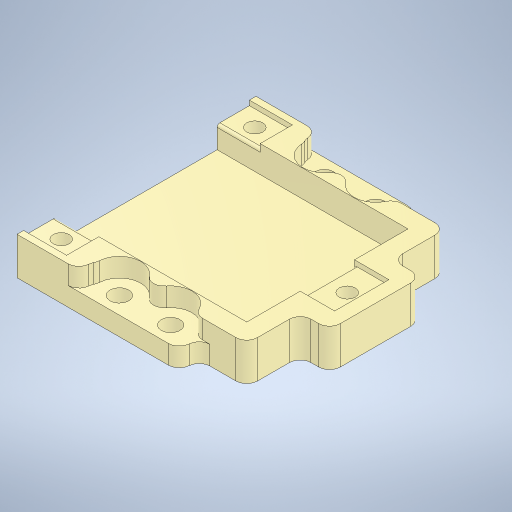
# Autodesk Inventor part: Servo Support
Saved by Autodesk Inventor 2023.2 (Build 272271000, 271)
## iProperties
Created: 2024-01-22
Part Number: Servo Support
Material: Nylon 6/6
Document SubType Name: Modeling
Designer: Nathan Cai
Density: 1.13 g/cm^3
Appearance: Nylon 6
Author: Nathan Cai
Autodesk Inventor part; units mm, degrees
ref_plane "YZ Plane" through (0, 0, 0) normal (1, 0, 0) x (0, 1, 0)
ref_plane "XZ Plane" through (0, 0, 0) normal (0, 1, 0) x (-1, 0, 0)
ref_plane "XY Plane" through (0, 0, 0) normal (0, 0, 1) x (1, 0, 0)
sketch "Sketch8" plane through (0, 0, 0) normal (0, 1, 0) x (-1, 0, 0)
  line L0 (-17.75, 15) -> (17.75, 15)
  line L1 (17.75, 15) -> (17.75, -15)
  line L2 (17.75, -15) -> (-17.75, -15)
  line L3 (-17.75, -15) -> (-17.75, 15)
  line L4 (-17.75, 15) -> (17.75, -15) construction
  line L5 (17.75, 15) -> (-17.75, -15) construction
  line L6 (17.75, 0) -> (-17.75, 0) construction
  line L7 (17.75, 21) -> (9.75, 21)
  line L8 (9.75, 21) -> (9.75, -21)
  line L9 (9.75, -21) -> (17.75, -21)
  line L10 (17.75, -21) -> (17.75, 21)
  line L11 (17.75, 21) -> (9.75, -21) construction
  line L12 (9.75, 21) -> (17.75, -21) construction
  line L13 (13.75, 21) -> (13.75, -21) construction
  circle A0 centre (13.75, 18) radius 1.5
  circle A1 centre (13.75, -18) radius 1.5
  line L14 (-24.15, 5.05) -> (-17.75, 5.05)
  line L15 (-17.75, 5.05) -> (-17.75, -5.05)
  line L16 (-17.75, -5.05) -> (-24.15, -5.05)
  line L17 (-24.15, -5.05) -> (-24.15, 5.05)
  line L18 (-24.15, 5.05) -> (-17.75, -5.05) construction
  line L19 (-17.75, 5.05) -> (-24.15, -5.05) construction
  circle A2 centre (-21.45, 0) radius 1.5
  line L20 (27.275, 14.4) -> (17.75, 14.4)
  line L21 (17.75, 14.4) -> (17.75, 2.4)
  line L22 (17.75, 2.4) -> (27.275, 2.4)
  line L23 (27.275, 2.4) -> (27.275, 14.4)
  line L24 (27.275, 14.4) -> (17.75, 2.4) construction
  line L25 (17.75, 14.4) -> (27.275, 2.4) construction
  line L26 (-26.7, 22.225) -> (17.75, 22.225)
  line L27 (17.75, 22.225) -> (17.75, -22.225)
  line L28 (17.75, -22.225) -> (-26.7, -22.225)
  line L29 (-26.7, -22.225) -> (-26.7, 22.225)
  line L30 (-26.7, 22.225) -> (17.75, -22.225) construction
  line L31 (17.75, 22.225) -> (-26.7, -22.225) construction
  point P0 (0, 0)
  point P1 (13.75, 0)
  point P2 (-20.95, 0)
  point P3 (22.5125, 8.4)
  point P4 (-4.475, 0)
  point P5 (9.75, -15)
  point P6 (9.75, 15)
  dimension "d120" = 35.5
  dimension "d121" = 30
  dimension "d122" = 8
  dimension "d123" = 42
  dimension "d124" = 3
  dimension "d126" = 41.9
  dimension "d127" = 10.1
  dimension "d128" = 36
  dimension "d129" = 3
  dimension "d130" = 35.2
  dimension "d131" = 9.6
  dimension "d132" = 12
  dimension "d133" = 9.525
  dimension "d134" = 44.45
  dimension "d135" = 44.45
  constraints: 64 end point, 14 midpoint, 10 parallel, 9 point on line, 5 horizontal, 5 perpendicular, 3 centre point, 1 symmetric about line, 1 other
  measures "d120" distance of L1.end L2.end
  measures "d121" distance of L0.end L1.end
  measures "d122" distance of L9.end L8.end
  measures "d123" distance of L8.end L7.end
  measures "d124" diameter of A0
  measures "d126" distance between parallel lines of L1 L17
  measures "d127" distance between parallel lines of L14 L16
  measures "d128" distance of A1.centre A0.centre
  measures "d129" diameter of A2
  measures "d130" distance from line of L13 A2.centre
  measures "d131" vertical distance of A0.centre point (22.512, 8.4)
  measures "d132" distance between parallel lines of L22 L20
  measures "d133" distance between parallel lines of L21 L23
  measures "d134" distance between parallel lines of L28 L26
  measures "d135" distance between parallel lines of L27 L29
extrude "Extrusion12" add sketch "Sketch8" against normal blind 7 contours L3 L14 L17 L16 L2 L8 L9 L27 L28 L29 L26 L7 L0 | L0 L8 L2 L3 | L8 L7 L10 L0 | L0 L1 L2 L8 | L3 L16 L17 L14 | L2 L10 L9 L8 | A0 | A1 | A2
extrude "Extrusion13" cut sketch "Sketch8" against normal blind 5 contours L0 L8 L2 L3 | L0 L1 L2 L8
extrude "Extrusion14" cut sketch "Sketch8" against normal blind 0.9 contours L8 L7 L10 L0 | L3 L16 L17 L14 | L2 L10 L9 L8 | A0 | A1 | A2
extrude "Extrusion15" cut sketch "Sketch8" against normal through all contours A0 | A1 | A2
shell "Shell1" thickness 3.5 removed faces 5 at (11.5667, 0, -19.4083) at (-2.9333, -2.3333, 22.225) at (-17.75, -6.3333, -5) at (26.7, -2.3333, 7.4083) at (11.8833, -2.3333, -22.225)
fillet "Fillet7" radius 0.5 5 edges at (-13.75, -0.9, -15) (17.75, -0.9, 0) (17.75, -0.9, 4.2065) (17.75, -0.9, -4.2065) (-13.75, -0.9, 15)
fillet "Fillet8" radius 2 10 edges at (-6.25, -1.75, 18.5) (21.25, -1.75, 18.5) (21.25, -1.75, 8.55) (21.25, -1.75, -8.55) (21.25, -1.75, -18.5) (-6.25, -1.75, -18.5) (26.7, -1.75, 8.55) (26.7, -1.75, -8.55) (-6.25, -1.75, 22.225) (-6.25, -1.75, -22.225)
sketch "Sketch9" plane through (0, 0, 0) normal (0, 1, 0) x (1, 0, 0)
  arc A0 (-6.2453, 20.3625) -> (-4.25, 18.5) centre (-4.25, 20.5) ccw projected
  line L0 (-4.25, 18.5) -> (19.25, 18.5) projected
  arc A1 (21.25, 16.5) -> (19.25, 18.5) centre (19.25, 16.5) ccw projected
  line L1 (21.25, 16.5) -> (21.25, 10.55) projected
  arc A2 (21.25, 10.55) -> (23.25, 8.55) centre (23.25, 10.55) ccw projected
  line L2 (23.25, 8.55) -> (24.7, 8.55) projected
  arc A3 (26.7, 6.55) -> (24.7, 8.55) centre (24.7, 6.55) ccw projected
  line L3 (26.7, 22.225) -> (26.7, 6.55) projected
  line L4 (-8.2405, 22.225) -> (26.7, 22.225) projected
  arc A4 (-6.2453, 20.3625) -> (-8.2405, 22.225) centre (-8.2405, 20.225) ccw projected
  arc A5 (23.25, -8.55) -> (21.25, -10.55) centre (23.25, -10.55) ccw projected
  line L5 (21.25, -10.55) -> (21.25, -16.5) projected
  arc A6 (19.25, -18.5) -> (21.25, -16.5) centre (19.25, -16.5) ccw projected
  line L6 (19.25, -18.5) -> (-4.25, -18.5) projected
  arc A7 (-4.25, -18.5) -> (-6.2453, -20.3625) centre (-4.25, -20.5) ccw projected
  arc A8 (-8.2405, -22.225) -> (-6.2453, -20.3625) centre (-8.2405, -20.225) ccw projected
  line L7 (26.7, -22.225) -> (-8.2405, -22.225) projected
  line L8 (26.7, -6.55) -> (26.7, -22.225) projected
  arc A9 (24.7, -8.55) -> (26.7, -6.55) centre (24.7, -6.55) ccw projected
  line L9 (24.7, -8.55) -> (23.25, -8.55) projected
  line L10 (-8.2405, 22.225) -> (26.7, 22.225) projected
  line L11 (26.7, -22.225) -> (-8.2405, -22.225) projected
  line L12 (26.7, 22.225) -> (12.4125, 22.225)
  line L13 (12.4125, 22.225) -> (12.4125, -22.225)
  line L14 (12.4125, -22.225) -> (26.7, -22.225)
  line L15 (26.7, -22.225) -> (26.7, 22.225)
  line L16 (26.7, 22.225) -> (26.7, 6.55) projected
  line L17 (26.7, 19.05) -> (-17.75, 19.05) construction
  line L18 (-17.75, 22.225) -> (-17.75, 21) projected
  line L19 (-17.75, -15) -> (-17.75, 15) projected
  line L20 (-17.75, 0) -> (26.7, 0) construction
  circle A10 centre (7.65, 19.05) radius 1.7526
  circle A11 centre (-1.875, 19.05) radius 1.7526
  circle A12 centre (7.65, -19.05) radius 1.7526
  circle A13 centre (-1.875, -19.05) radius 1.7526
  circle A14 centre (7.65, 19.05) radius 3.9688
  circle A15 centre (-1.875, 19.05) radius 3.9688
  circle A16 centre (7.65, -19.05) radius 3.9688
  circle A17 centre (-1.875, -19.05) radius 3.9688
  point P0 (0, 0)
  point P1 (12.4125, -18.5)
  point P2 (12.4125, -22.225)
  point P3 (12.4125, 18.5)
  dimension "d147" = 14.2875
  dimension "d148" = 19.05
  dimension "d149" = 3.5052
  dimension "d150" = 4.7625
  dimension "d153" = 9.525
  dimension "d161" = 7.9375
  dimension "d164" = 9.525
  constraints: 12 end point, 8 centre point, 4 point on line, 4 symmetric about line, 3 horizontal, 3 parallel, 2 midpoint, 1 coincident, 1 perpendicular, 8 other
  measures "d147" distance between parallel lines of L15 L13
  measures "d148" distance between parallel lines of L20 L17
  measures "d149" diameter of A10
  measures "d150" distance from line of L13 A10.centre
  measures "d153" distance of A10.centre A11.centre
  measures "d161" diameter of A14
  measures "d164" distance of A14.centre A15.centre
extrude "Extrusion16" cut sketch "Sketch9" against normal blind 10 contours A11 L0 | L0 A11 | A10 L0 | L0 A10 | L13 L4 L3 A3 L2 A2 L1 A1 L0 | L6 A6 L5 A5 L9 A9 L8 L7 L13 | A12 L6 | L6 A12 | A13 L6 | L6 A13
extrude "Extrusion17" cut sketch "Sketch9" against normal up to surface (3.5 mm away) contours A15 L4 L0 A11 A0 | A0 L0 A11 A15 | A15 L4 | A11 L0 | L0 A11 | A14 L4 L0 A10 | L0 A10 A14 | A14 L4 | A10 L0 | L0 A10 | A16 L7 L6 A12 | L6 A12 A16 | A12 L6 | L6 A12 | A16 L7 | A17 L7 A7 L6 A13 | L6 A13 A7 A17 | A13 L6 | L6 A13 | A17 L7
fillet "Fillet10" radius 2 12 edges at (-5.8369, -1.75, -19.2828) (2.0555, -1.75, -18.5) (3.7195, -1.75, -18.5) (12.4125, -5.25, -18.5) (12.4125, -5.25, -22.225) (11.5805, -1.75, -18.5) (12.4125, -5.25, 18.5) (12.4125, -5.25, 22.225) (11.5805, -1.75, 18.5) (3.7195, -1.75, 18.5) (2.0555, -1.75, 18.5) (-5.8369, -1.75, 19.2828)
chamfer "Chamfer4" distance 1.5 angle 45 3 edges at (-12.25, -7, 18) (22.95, -7, 0) (-12.25, -7, -18)
body "Solid3"
